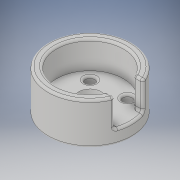
# Autodesk Inventor part: motor_mount
Saved by Autodesk Inventor 2019 (Build 230136000, 136)
## iProperties
Created: 2019-03-09
Part Number: motor_mount
Material: Generic
Document SubType Name: Modeling
Designer: Jaden
Density: 1 g/cm^3
Appearance: Default
Author: Jaden
Autodesk Inventor part; units mm, degrees
ref_plane "YZ Plane" through (0, 0, 0) normal (1, 0, 0) x (0, 1, 0)
ref_plane "XZ Plane" through (0, 0, 0) normal (0, 1, 0) x (-1, 0, 0)
ref_plane "XY Plane" through (0, 0, 0) normal (0, 0, 1) x (1, 0, 0)
sketch "Sketch1" plane through (0, 0, 0) normal (0, 1, 0) x (-1, 0, 0)
  circle A0 centre (0, 0) radius 12
  circle A1 centre (0, 0) radius 4
  circle A2 centre (0, 0) radius 15
  line L0 (-10.9087, -5) -> (-14.1421, -5)
  line L1 (-10.9087, 5) -> (-14.1421, 5)
  dimension "d0" = 5
  dimension "d2" = 10
  dimension "d3" = 8
  dimension "d4" = 30
  dimension "d5" = 3
  constraints: 4 end point, 4 point on circle, 3 centre point, 3 coincident, 2 horizontal
  measures "d0" distance from line of L0 point (0, 0)
  measures "d2" distance between parallel lines of L1 L0
  measures "d3" diameter of A1
  measures "d4" diameter of A2
  measures "d5" radial gap between concentric circles of A2 A0
extrude "Extrusion1" add sketch "Sketch1" along normal blind 15 contours A0 L1 A2 L0 picked at (13.8643, -1.1568)
sketch "Sketch2" plane through (0, 0, 0) normal (0, -1, 0) x (1, 0, 0)
  circle A0 centre (0, 0) radius 12
  circle A1 centre (0, 0) radius 4
  circle A2 centre (0, 0) radius 15
  line L0 (-10.9087, -5) -> (-14.1421, -5)
  line L1 (-10.9087, 5) -> (-14.1421, 5)
  dimension "d8" = 5
  dimension "d9" = 10
  dimension "d10" = 8
  dimension "d11" = 30
  dimension "d12" = 3
  constraints: 4 end point, 4 point on circle, 3 centre point, 3 coincident, 2 horizontal
  measures "d8" distance from line of L0 point (0, 0)
  measures "d9" distance between parallel lines of L1 L0
  measures "d10" diameter of A1
  measures "d11" diameter of A2
  measures "d12" radial gap between concentric circles of A2 A0
extrude "Extrusion2" add sketch "Sketch2" against normal blind 5 contours A0
sketch "Sketch3" plane through (0, 0, 0) normal (0, -1, 0) x (1, 0, 0)
  circle A0 centre (0, 0) radius 12
  circle A1 centre (0, 0) radius 4
  circle A2 centre (0, 0) radius 15
  line L0 (-10.9087, -5) -> (-14.1421, -5)
  line L1 (-10.9087, 5) -> (-14.1421, 5)
  dimension "d15" = 5
  dimension "d16" = 10
  dimension "d17" = 8
  dimension "d18" = 30
  dimension "d19" = 3
  constraints: 4 end point, 4 point on circle, 3 centre point, 3 coincident, 2 horizontal
  measures "d15" distance from line of L0 point (0, 0)
  measures "d16" distance between parallel lines of L1 L0
  measures "d17" diameter of A1
  measures "d18" diameter of A2
  measures "d19" radial gap between concentric circles of A2 A0
extrude "Extrusion3" add sketch "Sketch3" against normal blind 5 contours A0 L1 A2 L0 picked at (13.8643, -1.1568)
sketch "Sketch4" plane through (0, 0, 0) normal (0, -1, 0) x (1, 0, 0)
  circle A0 centre (0, 0) radius 12
  circle A1 centre (0, 0) radius 4
  circle A2 centre (0, 0) radius 15
  line L0 (-10.9087, -5) -> (-14.1421, -5)
  line L1 (-10.9087, 5) -> (-14.1421, 5)
  dimension "d22" = 5
  dimension "d23" = 10
  dimension "d24" = 8
  dimension "d25" = 30
  dimension "d26" = 3
  constraints: 4 end point, 4 point on circle, 3 centre point, 3 coincident, 2 horizontal
  measures "d22" distance from line of L0 point (0, 0)
  measures "d23" distance between parallel lines of L1 L0
  measures "d24" diameter of A1
  measures "d25" diameter of A2
  measures "d26" radial gap between concentric circles of A2 A0
extrude "Extrusion4" add sketch "Sketch4" against normal blind 2 contours A1
sketch "Sketch5" plane through (0, 0, 0) normal (0, -1, 0) x (1, 0, 0)
  circle A0 centre (-6.7175, 6.7175) radius 1.7
  circle A1 centre (5.6568, 5.6568) radius 1.7
  circle A2 centre (6.7175, -6.7175) radius 1.7
  circle A3 centre (-5.6569, -5.6569) radius 1.7
  line L0 (0, 0) -> (-10.6066, 10.6066) construction
  arc A4 (14.1421, 5) -> (14.1421, -5) centre (0, 0) ccw projected
  line L1 (0, 0) -> (15, 0) construction
  line L2 (0, 0) -> (10.6066, -10.6066) construction
  line L3 (0, 0) -> (15, 0) construction
  line L4 (0, 0) -> (-10.6066, -10.6066) construction
  line L5 (0, 0) -> (10.6066, 10.6066) construction
  line L6 (0, 0) -> (15, 0) construction
  dimension "d29" = 3.4
  dimension "d30" = 3.4
  dimension "d31" = 3.4
  dimension "d32" = 3.4
  dimension "d34" = 135
  dimension "d35" = 45
  dimension "d36" = 45
  dimension "d37" = 11.3137
  dimension "d38" = 5.6569
  dimension "d39" = 13.435
  dimension "d41" = 6.7175
  constraints: 14 end point, 4 centre point, 4 point on circle, 4 point on line, 3 equal length, 3 horizontal, 1 perpendicular
  measures "d29" diameter of A0
  measures "d30" diameter of A1
  measures "d31" diameter of A2
  measures "d32" diameter of A3
  measures "d34" angle of L1 L0
  measures "d35" angle of L2 L3
  measures "d36" angle of L6 L5
  measures "d37" horizontal distance of A3.centre A1.centre
  measures "d38" horizontal distance of L0.start A3.centre
  measures "d39" horizontal distance of A0.centre A2.centre
  measures "d41" horizontal distance of A0.centre L0.start
extrude "Extrusion5" cut sketch "Sketch5" against normal through all
fillet "Fillet1" radius 0.7937 12 edges at (-12, 15, 0) (-15, 15, 0) (12.5254, 15, 5) (14.1421, 10, 5) (15, 5, 0) (14.1421, 10, -5) (12.5254, 15, -5) (12.5254, 5, -5) (12.5254, 5, 5) (10.9087, 10, 5) (10.9087, 10, -5) (-14.1421, 0, 5)
fillet "Fillet2" radius 0.7937 8 edges at (3.9568, 0, 5.6568) (5.0175, 0, -6.7175) (-7.3569, 0, -5.6569) (-8.4175, 0, 6.7175) (-8.4175, 5, 6.7175) (-7.3569, 5, -5.6569) (3.9568, 5, 5.6568) (5.0175, 5, -6.7175)
body "Solid1"
